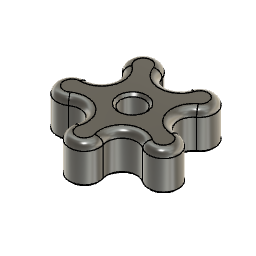
Knob_v0.1 (Autodesk Fusion 360 design; units mm, degrees)
Autodesk Fusion 360 part; units mm, degrees
sketch "Sketch1" plane through (0, 0, 0) normal (0, 0, 1) x (1, 0, 0)
  circle A0 centre (0, 0) radius 31.6631 construction
  circle A1 centre (0, 31.6631) radius 21.7092 construction
  circle A2 centre (27.4211, -15.8316) radius 21.7092 construction
  circle A3 centre (-27.4211, -15.8316) radius 21.7092 construction
  line L0 (0, 0) -> (0, 31.6631) construction
  line L1 (0, 0) -> (27.4211, -15.8316) construction
  line L2 (0, 0) -> (-27.4211, -15.8316) construction
  circle A4 centre (2.3751, -0.3675) radius 18.8772 construction
  circle A5 centre (0, -19.0946) radius 5.9054
  circle A6 centre (0, 0) radius 25 construction
  circle A7 centre (0, 0) radius 4.65
  line L3 (0, 0) -> (0, -19.0946) construction
  line L4 (0, 0) -> (-16.4545, 9.5) construction
  line L5 (0, 0) -> (6.5253, -3.7674)
  circle A8 centre (18.1601, -5.9006) radius 5.9054
  circle A9 centre (11.2236, 15.4479) radius 5.9054
  circle A10 centre (-11.2236, 15.4479) radius 5.9054
  circle A11 centre (-18.1601, -5.9006) radius 5.9054
  arc A12 (14.7009, -10.6867) -> (5.6208, -17.2837) centre (11.2417, -15.4728) ccw
  arc A13 (14.7065, 10.679) -> (18.1748, 0.0048) centre (18.1894, 5.9101) ccw
  arc A14 (-5.6118, 17.2867) -> (5.6118, 17.2867) centre (0, 19.1255) ccw
  arc A15 (-18.1748, 0.0048) -> (-14.7065, 10.679) centre (-18.1894, 5.9101) ccw
  arc A16 (-5.6208, -17.2837) -> (-14.7009, -10.6867) centre (-11.2417, -15.4728) ccw
  dimension "d1" = 120
  dimension "d4" = 50
  dimension "d6" = 9.3
  dimension "d21" = 50
  dimension "d22" = 360
  dimension "d23" = 50
  dimension "d24" = 360
  constraint coincident A0.centre L0.start
  constraint coincident A0 A1.centre
  constraint coincident A0 A2.centre
  constraint coincident A0 A3.centre
  constraint equal A1 A2
  constraint equal A2 A3
  constraint coincident A1.centre L0.end
  constraint vertical L0
  constraint coincident A2.centre L1.end
  constraint coincident A3.centre L2.end
  constraint coincident A4 A5.centre
  constraint tangent A3 A5
  constraint tangent A2 A5
  constraint coincident A5.centre L3.end
  constraint coincident L1 L5.end
  constraint vertical L3
  constraint tangent A5 A6
  constraint coincident A8 A12.start
  constraint coincident A5 A12.end
  constraint tangent A8 A12
  constraint tangent A5 A12
  constraint equal A5 A12
  measures "d1" angle of L0 L2
  measures "d4" diameter of A6
  measures "d6" diameter of A7
extrude "Extrude1" add sketch "Sketch1" along normal blind 15
fillet "Fillet1" radius 2.717 10 edges at (7.7706, -10.6953, 15) (23.7764, -7.7254, 15) (12.5731, 4.0852, 15) (14.6946, 20.2254, 15) (0, 13.2201, 15) (-14.6946, 20.2254, 15) (-12.5731, 4.0852, 15) (-23.7764, -7.7254, 15) (-7.7706, -10.6953, 15) (0, -25, 15)
chamfer "Chamfer3" distance 0.8 angle 45 11 edges at (7.7706, -10.6953, 0) (23.7764, -7.7254, 0) (12.5731, 4.0852, 0) (14.6946, 20.2254, 0) (0, 13.2201, 0) (-14.6946, 20.2254, 0) (-12.5731, 4.0852, 0) (-23.7764, -7.7254, 0) (-7.7706, -10.6953, 0) (0, -25, 0) (-4.3353, 1.6815, 0)
chamfer "Chamfer4" distance 1 angle 45 1 edges at (-4.3353, 1.6815, 15)
